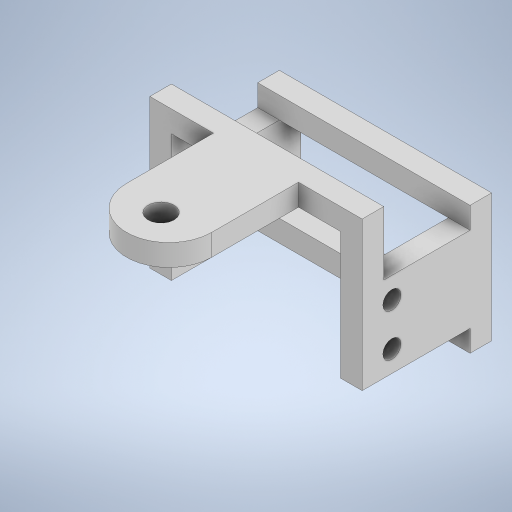
# Autodesk Inventor part: Part2_cage
Saved by Autodesk Inventor 2024 (Build 280153000, 153)
## iProperties
Created: 2023-06-11
Part Number: Part2_cage
Material: Generic
Document SubType Name: Modeling
Designer: abhin
Density: 1 g/cm^3
Appearance: Default
Author: abhin
Autodesk Inventor part; units mm, degrees
ref_plane "YZ Plane" through (0, 0, 0) normal (1, 0, 0) x (0, 1, 0)
ref_plane "XZ Plane" through (0, 0, 0) normal (0, 1, 0) x (-1, 0, 0)
ref_plane "XY Plane" through (0, 0, 0) normal (0, 0, 1) x (1, 0, 0)
sketch "Sketch1" plane through (0, 0, 0) normal (0, 0, 1) x (1, 0, 0)
  line L0 (-19.603, -9.85) -> (19.603, -9.85)
  line L1 (19.603, -9.85) -> (19.603, 9.85)
  line L2 (19.603, 9.85) -> (-19.603, 9.85)
  line L3 (-19.603, 9.85) -> (-19.603, -9.85)
  line L4 (-19.603, -9.85) -> (19.603, 9.85) construction
  line L5 (19.603, -9.85) -> (-19.603, 9.85) construction
  line L6 (-24.603, 14.85) -> (24.603, 14.85)
  line L7 (24.603, 14.85) -> (24.603, -14.85)
  line L8 (24.603, -14.85) -> (-24.603, -14.85)
  line L9 (-24.603, -14.85) -> (-24.603, 14.85)
  point P0 (0, 0)
  dimension "d0" = 39.206
  dimension "d1" = 19.7
  dimension "d2" = 5
  constraints: 20 end point, 4 parallel, 2 midpoint, 2 perpendicular, 1 horizontal, 3 other
  measures "d0" distance of L2.end L1.end
  measures "d1" distance of L1.end L0.end
  measures "d2" distance between parallel lines of L2 L6
extrude "Extrusion1" add sketch "Sketch1" along normal blind 5
sketch "Sketch2" plane through (0, 0, 5) normal (0, 0, 1) x (1, 0, 0)
  line L0 (-24.603, 14.85) -> (-24.603, -14.85) construction
  line L1 (-24.603, 14.85) -> (-24.603, -14.85) construction
  line L2 (24.603, 14.85) -> (-24.603, 14.85) construction
  line L3 (-24.603, 14.85) -> (24.603, 14.85) construction
  line L4 (24.603, -14.85) -> (24.603, 14.85) construction
  line L5 (24.603, 14.85) -> (24.603, -14.85) construction
  line L6 (24.603, -14.85) -> (-24.603, -14.85) construction
  line L7 (-19.603, -9.85) -> (-19.603, 9.85) projected
  line L8 (-19.603, 9.85) -> (-24.603, 9.85)
  line L9 (-24.603, 9.85) -> (-24.603, -9.85)
  line L10 (-24.603, -9.85) -> (-19.603, -9.85)
  line L11 (-19.603, -9.85) -> (-19.603, 9.85)
  line L12 (19.603, 9.85) -> (19.603, -9.85) projected
  line L13 (19.603, 9.85) -> (24.603, 9.85)
  line L14 (24.603, 9.85) -> (24.603, -9.85)
  line L15 (24.603, -9.85) -> (19.603, -9.85)
  line L16 (19.603, -9.85) -> (19.603, 9.85)
  point P0 (0, 0)
  constraints: 24 end point, 6 equal length, 4 perpendicular, 3 point on line, 2 horizontal
extrude "Extrusion2" add sketch "Sketch2" along normal blind 25
sketch "Sketch3" plane through (0, 0, 0) normal (1, 0, 0) x (0, 1, 0)
  circle A0 centre (4.925, 23.111) radius 2.1
  line L0 (14.85, 0) -> (14.85, 5) projected
  line L1 (14.85, 5) -> (9.85, 5) projected
  circle A1 centre (-4.925, 23.111) radius 2.1
  line L2 (-14.85, 0) -> (-14.85, 5) projected
  line L3 (-9.85, 5) -> (-14.85, 5) projected
  point P0 (0, 0)
  point P1 (-12.35, 5)
  dimension "d7" = 4.2
  dimension "d8" = 9.925
  dimension "d9" = 18.111
  dimension "d10" = 4.2
  dimension "d11" = 9.925
  dimension "d12" = 18.111
  constraints: 2 centre point, 1 midpoint
  measures "d7" diameter of A0
  measures "d8" distance from line of L0 A0.centre
  measures "d9" distance from line of L1 A0.centre
  measures "d10" diameter of A1
  measures "d11" distance from line of L2 A1.centre
  measures "d12" vertical distance of point (-12.35, 5) A1.centre
extrude "Extrusion3" cut sketch "Sketch3" along normal through all both and the other way through all
sketch "Sketch4" plane through (0, 0, 0) normal (1, 0, 0) x (0, 1, 0)
  line L0 (-9.85, 30) -> (9.85, 30) construction
  line L1 (0, 30) -> (0, 0) construction
  line L2 (24.603, 30) -> (19.603, 30)
  line L3 (19.603, 30) -> (19.603, 25)
  line L4 (19.603, 25) -> (24.603, 25)
  line L5 (24.603, 25) -> (24.603, 30)
  line L6 (14.85, 0) -> (-14.85, 0) projected
  point P0 (19.603, 27.5)
  dimension "d29" = 5
  dimension "d30" = 5
  dimension "d31" = 19.603
  dimension "d32" = 25
  constraints: 10 end point, 2 midpoint, 2 parallel, 1 horizontal, 1 perpendicular, 1 vertical
  measures "d29" distance of L4.end L3.end
  measures "d30" distance of L3.end L2.end
  measures "d31" distance from line of L1 point (19.603, 27.5)
  measures "d32" distance between parallel lines of L6 L4
extrude "Extrusion4" add sketch "Sketch4" along normal mid plane 49.206
sketch "Sketch5" plane through (0, 0, 30) normal (0, 0, 1) x (1, 0, 0)
  line L0 (-24.603, -9.85) -> (-24.603, 14.85) projected
  line L1 (24.603, -9.85) -> (24.603, 14.85) projected
  line L2 (-24.603, 24.603) -> (24.603, 24.603) projected
  line L3 (-9.85, 24.603) -> (9.85, 24.603)
  line L4 (9.85, 24.603) -> (9.85, 19.603)
  line L5 (9.85, 19.603) -> (-9.85, 19.603)
  line L6 (-9.85, 19.603) -> (-9.85, 24.603)
  line L7 (24.603, 24.603) -> (24.603, 19.603) projected
  line L8 (-24.603, 19.603) -> (-24.603, 24.603) projected
  point P0 (0, 0)
  point P1 (9.85, 22.103)
  point P2 (-24.603, 22.103)
  point P3 (9.85, 24.603)
  dimension "d33" = 19.7
  dimension "d34" = 5
  dimension "d35" = 14.753
  dimension "d36" = 14.753
  constraints: 8 end point, 2 midpoint, 2 parallel, 1 horizontal, 1 perpendicular, 1 point on line
  measures "d33" distance of L4.end L5.end
  measures "d34" distance of L3.end L4.end
  measures "d35" distance from line of L7 point (9.85, 22.103)
  measures "d36" distance from line of L6 point (-24.603, 22.103)
extrude "Extrusion5" add sketch "Sketch5" along normal blind 30
sketch "Sketch7" plane through (19.603, 9.85, 5) normal (0, 1, 0) x (1, 0, 0)
  line L0 (-39.206, 0) -> (-39.206, -25) projected
  line L1 (-39.206, -25) -> (-44.206, -25)
  line L2 (-44.206, -25) -> (-44.206, -20)
  line L3 (-44.206, -20) -> (-39.206, -20)
  line L4 (-39.206, -20) -> (-39.206, -25)
  line L5 (0, 0) -> (0, -25) projected
  line L6 (0, -25) -> (5, -25)
  line L7 (5, -25) -> (5, -20)
  line L8 (5, -20) -> (0, -20)
  line L9 (0, -20) -> (0, -25)
  point P0 (-19.603, 5)
  dimension "d37" = 5
  dimension "d38" = 5
  dimension "d39" = 5
  dimension "d40" = 5
  constraints: 16 end point, 4 parallel, 2 horizontal, 2 perpendicular
  measures "d37" distance of L2.end L3.end
  measures "d38" distance of L1.end L2.end
  measures "d39" distance of L8.end L7.end
  measures "d40" distance of L7.end L6.end
extrude "Extrusion7" add sketch "Sketch7" along normal through all
sketch "Sketch8" plane through (-24.603, 24.603, 25) normal (0, 1, 0) x (1, 0, 0)
  line L0 (14.753, -35) -> (34.453, -35) construction
  line L1 (24.603, -35) -> (24.603, 0) construction
  line L2 (5, 0) -> (44.206, 0) construction
  circle A0 centre (24.603, -27) radius 3
  point P0 (24.603, 25)
  dimension "d43" = 6
  dimension "d44" = 8
  constraints: 2 end point, 2 midpoint, 1 centre point, 1 point on line
  measures "d43" diameter of A0
  measures "d44" distance from line of A0.centre L0
extrude "Extrusion8" cut sketch "Sketch8" against normal through all
fillet "Fillet1" radius 9.85 2 edges at (9.85, 22.103, 60) (-9.85, 22.103, 60)
body "Solid1"
